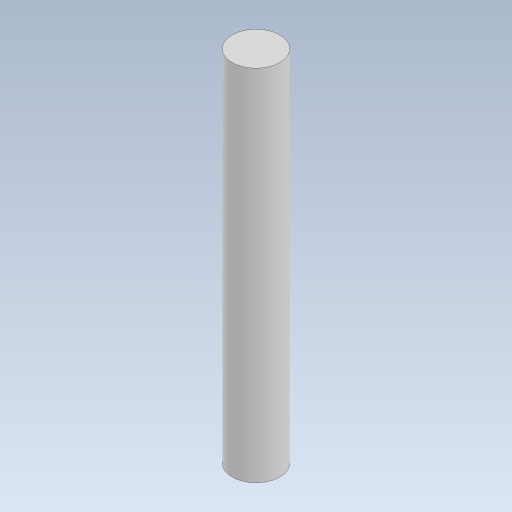
# Autodesk Inventor part: axle 4_30
Saved by Autodesk Inventor 2023 (Build 270158000, 158)
## iProperties
Created: 2023-03-17
Part Number: axle 4_30
Material: 壓克力條
Document SubType Name: Modeling
Designer: JOU
Density: 0.9185 g/cm^3
Appearance: 預設
Mass: 0.230844 g
Surface Area: 2.7646 cm^2
Volume: 0.251327 cm^3
Author: JOU
Title: 壓克力軸
Autodesk Inventor part; units mm, degrees
ref_plane "YZ Plane" through (0, 0, 0) normal (1, 0, 0) x (0, 1, 0)
ref_plane "XZ Plane" through (0, 0, 0) normal (0, 1, 0) x (-1, 0, 0)
ref_plane "XY Plane" through (0, 0, 0) normal (0, 0, 1) x (1, 0, 0)
sketch "草圖1" plane through (0, 0, 0) normal (0, 1, 0) x (-1, 0, 0)
  circle A0 centre (0, 0) radius 2
  dimension "d0" = 4
  constraints: 1 centre point, 1 coincident
  measures "d0" diameter of A0
extrude "擠出1" add sketch "草圖1" along normal blind 30
